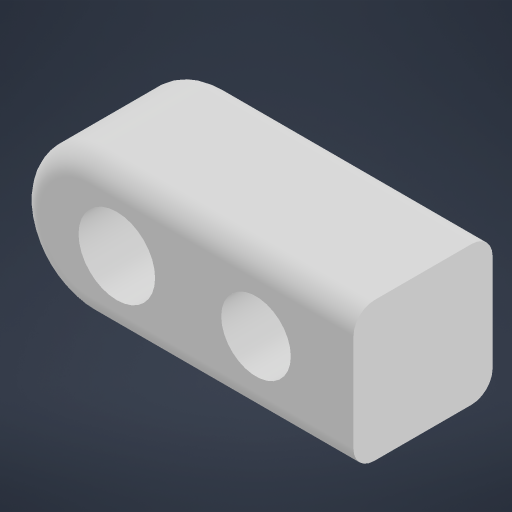
# Autodesk Inventor part: Hole_TestFits
Saved by Autodesk Inventor 2024 (Build 280153000, 153)
## iProperties
Created: 2023-07-01
Part Number: Hole_TestFits
Material: Generic
Document SubType Name: Modeling
Designer: User
Density: 1 g/cm^3
Appearance: Default
Author: User
Autodesk Inventor part; units mm, degrees
ref_plane "YZ Plane" through (0, 0, 0) normal (1, 0, 0) x (0, 1, 0)
ref_plane "XZ Plane" through (0, 0, 0) normal (0, 1, 0) x (-1, 0, 0)
ref_plane "XY Plane" through (0, 0, 0) normal (0, 0, 1) x (1, 0, 0)
sketch "Sketch8" plane through (0, 0, 0) normal (0, 0, 1) x (1, 0, 0)
  line L0 (0, 0) -> (-10, 0)
  line L1 (-10, 0) -> (-10, 10)
  line L2 (-10, 10) -> (0, 10)
  line L3 (0, 10) -> (0, 0)
  dimension "d38" = 10
  dimension "d39" = 10
  constraints: 8 end point, 2 parallel, 1 horizontal, 1 perpendicular
  measures "d38" distance of L1.end L2.end
  measures "d39" distance of L0.end L1.end
extrude "Extrusion5" add sketch "Sketch8" along normal blind 10
sketch "Sketch9" plane through (0, 0, 10) normal (0, 0, 1) x (1, 0, 0)
  point P0 (0, 0)
  point P1 (-5, 5)
hole "Hole3" at (-5, 5, 10) direction (0, 0, -1) diameter 4 depth 10 counterbore diameter 5.5 counterbore depth 5
sketch "Sketch14" plane through (-10, 0, 0) normal (-1, 0, 0) x (0, 0, 1)
  line L0 (0, 0) -> (10, 0)
  line L1 (10, 0) -> (10, 10)
  line L2 (10, 10) -> (0, 10)
  line L3 (0, 10) -> (0, 0)
  dimension "d71" = 10
  dimension "d72" = 10
  constraints: 8 end point, 2 parallel, 1 horizontal, 1 perpendicular
  measures "d71" distance of L2.end L1.end
  measures "d72" distance of L1.end L0.end
extrude "Extrusion9" add sketch "Sketch14" along normal blind 2
fillet "Fillet1" radius 5 2 edges at (-12, 10, 5) (-12, 0, 5)
sketch "Sketch15" plane through (0, 0, 0) normal (1, 0, 0) x (0, 0, -1)
  line L0 (-10, 0) -> (-10, 10) projected
  line L1 (0, 0) -> (-10, 0)
  line L2 (-10, 0) -> (-10, 10)
  line L3 (-10, 10) -> (0, 10)
  line L4 (0, 10) -> (0, 0)
  dimension "d76" = 10
  dimension "d77" = 10
  constraints: 8 end point, 2 parallel, 1 horizontal, 1 perpendicular
  measures "d76" distance of L0.end L3.end
  measures "d77" distance of L1.end L0.end
extrude "Extrusion10" add sketch "Sketch15" along normal blind 10
sketch "Sketch16" plane through (0, 0, 10) normal (0, 0, 1) x (1, 0, 0)
  point P0 (0, 0)
  point P1 (5, 5)
hole "Hole5" at (5, 5, 10) direction (0, 0, -1) diameter 4 depth 10 counterbore diameter 5 counterbore depth 4.5
sketch "Sketch17" plane through (10, 0, 0) normal (1, 0, 0) x (0, 0, -1)
  line L0 (0, 0) -> (-10, 0)
  line L1 (-10, 0) -> (-10, 10)
  line L2 (-10, 10) -> (0, 10)
  line L3 (0, 10) -> (0, 0)
  dimension "d87" = 10
  dimension "d88" = 10
  constraints: 8 end point, 2 parallel, 1 horizontal, 1 perpendicular
  measures "d87" distance of L1.end L2.end
  measures "d88" distance of L0.end L1.end
extrude "Extrusion11" add sketch "Sketch17" along normal blind 2
fillet "Fillet2" radius 1.5 6 edges at (-10.5357, 8.5357, 10) (2.4997, 0, 10) (2.4998, 10, 10) (-10.5357, 8.5357, 0) (2.4997, 0, 0) (2.4998, 10, 0)
body "Solid3"
